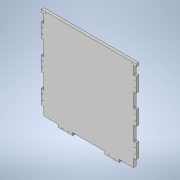
# Autodesk Inventor part: bottom-tool_part
Saved by Autodesk Inventor 2020 (Build 240168000, 168)
## iProperties
Created: 2019-12-17
Part Number: bottom-tool_part
Material: Generic
Document SubType Name: Modeling
Designer: fabfarm
Density: 1 g/cm^3
Appearance: Default
Author: fabfarm
Autodesk Inventor part; units mm, degrees
ref_plane "YZ Plane" through (0, 0, 0) normal (1, 0, 0) x (0, 1, 0)
ref_plane "XZ Plane" through (0, 0, 0) normal (0, 1, 0) x (-1, 0, 0)
ref_plane "XY Plane" through (0, 0, 0) normal (0, 0, 1) x (1, 0, 0)
sketch "Sketch1" plane through (0, 0, 0) normal (0, 0, 1) x (1, 0, 0)
  line L0 (330, -307.45) -> (-330, -307.45)
  line L1 (-330, -307.45) -> (-330, 307.45)
  line L2 (-330, 307.45) -> (330, 307.45)
  line L3 (330, 307.45) -> (330, -307.45)
  line L4 (330, -307.45) -> (-330, 307.45) construction
  line L5 (-330, -307.45) -> (330, 307.45) construction
  point P0 (0, 0)
  dimension "d0" = 614.9
  dimension "d1" = 660
  constraints: 12 end point, 2 midpoint, 2 parallel, 1 horizontal, 1 perpendicular
  measures "d0" distance of L2.end L0.start
  measures "d1" distance of L0.start L0.end
extrude "Extrusion1" add sketch "Sketch1" along normal blind 18.55
sketch "Sketch2" plane through (0, 0, 18.55) normal (0, 0, 1) x (1, 0, 0)
  line L0 (-330, 307.45) -> (-330, -307.45) construction
  line L1 (330, 307.45) -> (-330, 307.45) construction
  line L2 (-330, 307.45) -> (-311.45, 307.45)
  line L3 (-311.45, 307.45) -> (-311.45, 250)
  line L4 (-311.45, 250) -> (-330, 250)
  line L5 (-330, 250) -> (-330, 307.45)
  line L6 (-330, -307.45) -> (330, -307.45) projected
  line L7 (-330, -307.45) -> (-311.45, -307.45)
  line L8 (-311.45, -307.45) -> (-311.45, -250)
  line L9 (-311.45, -250) -> (-330, -250)
  line L10 (-330, -250) -> (-330, -307.45)
  line L11 (-330, -150) -> (-311.45, -150)
  line L12 (-311.45, -150) -> (-311.45, -50)
  line L13 (-311.45, -50) -> (-330, -50)
  line L14 (-330, -50) -> (-330, -150)
  line L15 (-330, 50) -> (-311.45, 50)
  line L16 (-311.45, 50) -> (-311.45, 150)
  line L17 (-311.45, 150) -> (-330, 150)
  line L18 (-330, 150) -> (-330, 50)
  point P0 (0, 0)
  dimension "d21" = 100
  dimension "d22" = 100
  dimension "d23" = 100
  dimension "d24" = 100
  dimension "d25" = 57.45
  dimension "d26" = 18.55
  dimension "d30" = 100
  constraints: 32 end point, 8 parallel, 5 point on line, 4 horizontal, 4 perpendicular, 3 collinear
  measures "d21" distance between parallel lines of L4 L17
  measures "d22" distance of L15.end L16.end
  measures "d23" distance between parallel lines of L13 L15
  measures "d24" distance of L11.end L12.end
  measures "d25" distance of L2.end L3.end
  measures "d26" distance of L0.end L7.end
  measures "d30" distance between parallel lines of L11 L9
extrude "Extrusion2" cut sketch "Sketch2" against normal blind 18.55
mirror "Mirror1" about plane through (0, 0, 0) normal (1, 0, 0) of "Extrusion2"
sketch "Esquisse5" plane through (0, 0, 18.55) normal (0, 0, 1) x (1, 0, 0)
  circle A0 centre (-312.5743, 251.1243) radius 1.59
  circle A1 centre (-312.5743, 148.8757) radius 1.59
  circle A2 centre (-312.5743, 51.1243) radius 1.59
  circle A3 centre (-312.5743, -51.1243) radius 1.59
  circle A4 centre (-312.5743, -148.8757) radius 1.59
  circle A5 centre (-312.5743, -251.1243) radius 1.59
  line L0 (311.45, 307.45) -> (-311.45, 307.45) projected
  line L1 (0, 307.45) -> (0, -307.45) construction
  line L2 (-311.45, -307.45) -> (311.45, -307.45) projected
  circle A6 centre (312.5743, 251.1243) radius 1.59
  circle A7 centre (312.5743, 148.8757) radius 1.59
  circle A8 centre (312.5743, 51.1243) radius 1.59
  circle A9 centre (312.5743, -51.1243) radius 1.59
  circle A10 centre (312.5743, -148.8757) radius 1.59
  circle A11 centre (312.5743, -251.1243) radius 1.59
  line L3 (-312.5743, 251.1243) -> (-311.45, 250) construction
  line L4 (-311.45, 250) -> (-330, 250) projected
  point P0 (0, 0)
  point P1 (-330, 50)
  point P2 (-330, -50)
  point P3 (-311.45, -250)
  point P4 (-311.45, -150)
  point P5 (-311.45, -50)
  point P6 (-311.45, 50)
  point P7 (-311.45, 150)
  dimension "d27" = 3.18
  dimension "d57" = 45
  constraints: 6 centre point, 6 symmetric about line, 5 vertical alignment, 4 end point, 2 midpoint, 24 other
  measures "d57" angle of L3 L4
extrude "Extrusion5" cut sketch "Esquisse5" against normal blind 18.55
sketch "Esquisse7" plane through (0, 0, 18.55) normal (0, 0, 1) x (1, 0, 0)
  line L0 (-311.45, -307.45) -> (311.45, -307.45) projected
  line L1 (-211.45, -307.45) -> (-111.45, -307.45)
  line L2 (-111.45, -307.45) -> (-111.45, -326)
  line L3 (-111.45, -326) -> (-211.45, -326)
  line L4 (-211.45, -326) -> (-211.45, -307.45)
  line L5 (111.55, -307.45) -> (211.45, -307.45)
  line L6 (211.45, -307.45) -> (211.45, -326)
  line L7 (211.45, -326) -> (111.55, -326)
  line L8 (111.55, -326) -> (111.55, -307.45)
  line L9 (-311.45, -252.2486) -> (-311.45, -307.45) projected
  line L10 (311.45, -307.45) -> (311.45, -252.2486) projected
  line L11 (-330, 50) -> (-330, -50) projected
  line L12 (-330, 0) -> (330, 0) construction
  line L13 (330, -50) -> (330, 50) projected
  circle A0 centre (-181.45, -316.725) radius 2.25
  circle A1 centre (-141.45, -316.725) radius 2.25
  circle A2 centre (141.55, -316.725) radius 2.25
  circle A3 centre (181.45, -316.725) radius 2.25
  line L14 (-211.45, -316.725) -> (-111.45, -316.725) construction
  line L15 (311.45, 307.45) -> (-311.45, 307.45) projected
  line L16 (-311.45, 307.45) -> (311.45, 307.45)
  line L17 (311.45, 307.45) -> (311.45, 326)
  line L18 (311.45, 326) -> (-311.45, 326)
  line L19 (-311.45, 326) -> (-311.45, 307.45)
  line L20 (311.45, 252.2486) -> (311.45, 307.45) projected
  point P0 (0, 0)
  point P1 (-111.45, -307.45)
  dimension "d41" = 100
  dimension "d42" = 99.9
  dimension "d43" = 100
  dimension "d44" = 100
  dimension "d45" = 18.55
  dimension "d46" = 4.5
  dimension "d47" = 30
  dimension "d48" = 30
  dimension "d49" = 30
  dimension "d50" = 30
  dimension "d56" = 18.55
  constraints: 28 end point, 7 point on line, 6 parallel, 4 centre point, 4 midpoint, 3 equal radius, 3 horizontal, 3 perpendicular, 1 collinear
  measures "d41" distance of L2.end L3.end
  measures "d42" distance of L6.end L7.end
  measures "d43" distance between parallel lines of L9 L4
  measures "d44" distance between parallel lines of L6 L10
  measures "d45" distance of L1.end L2.end
  measures "d46" diameter of A0
  measures "d47" distance from line of L4 A0.centre
  measures "d48" distance from line of L2 A1.centre
  measures "d49" distance from line of L8 A2.centre
  measures "d50" distance from line of L6 A3.centre
  measures "d56" distance between parallel lines of L18 L15
extrude "Extrusion7" add sketch "Esquisse7" against normal blind 18.55
sketch "Esquisse6" plane through (0, 0, 18.55) normal (0, 0, 1) x (1, 0, 0)
  line L0 (-321.8493, -50) -> (-321.8493, 50) construction
  line L1 (-313.6986, 50) -> (-330, 50) construction
  line L2 (-313.6986, 150) -> (-330, 150) construction
  line L3 (-313.6986, 250) -> (-330, 250) construction
  circle A0 centre (-321.8493, 220) radius 2.25
  line L4 (-330, -50) -> (-313.6986, -50) projected
  line L5 (-0.195, -446.756) -> (0, 307.45) construction
  line L6 (311.45, 307.45) -> (-311.45, 307.45) projected
  line L7 (-321.8493, 150) -> (-321.8493, 250) construction
  circle A1 centre (-321.8493, 180) radius 2.25
  circle A2 centre (-321.8493, 20) radius 2.25
  circle A3 centre (-321.8493, -20) radius 2.25
  line L8 (-313.6986, -150) -> (-330, -150) projected
  line L9 (-321.8493, -150) -> (-321.8493, -250) construction
  line L10 (-313.6986, -250) -> (-330, -250) projected
  circle A4 centre (-321.8493, -180) radius 2.25
  circle A5 centre (-321.8493, -220) radius 2.25
  line L11 (321.6645, -50.1663) -> (321.7162, 49.8336) construction
  line L12 (313.5655, 49.8379) -> (329.8669, 49.8294) construction
  line L13 (313.6172, 149.8378) -> (329.9186, 149.8294) construction
  line L14 (313.6689, 249.8378) -> (329.9703, 249.8294) construction
  circle A6 centre (321.804, 219.8336) radius 2.25
  line L15 (329.8152, -50.1706) -> (313.5138, -50.1621)
  line L16 (321.7679, 149.8336) -> (321.8196, 249.8336) construction
  circle A7 centre (321.7834, 179.8336) radius 2.25
  circle A8 centre (321.7007, 19.8336) radius 2.25
  circle A9 centre (321.68, -20.1663) radius 2.25
  line L17 (313.4621, -150.1621) -> (329.7635, -150.1705)
  line L18 (321.6128, -150.1663) -> (321.5611, -250.1663) construction
  line L19 (313.4104, -250.1621) -> (329.7118, -250.1705)
  circle A10 centre (321.5973, -180.1663) radius 2.25
  circle A11 centre (321.5766, -220.1663) radius 2.25
  point P0 (0, 0)
  dimension "d34" = 30
  dimension "d35" = 30
  dimension "d36" = 30
  dimension "d37" = 30
  dimension "d38" = 4.5
  dimension "d39" = 30
  dimension "d40" = 30
  constraints: 26 end point, 24 symmetric about line, 12 centre point, 12 point on line, 8 midpoint, 5 equal radius, 1 vertical, 6 other
  measures "d34" distance from line of L3 A0.centre
  measures "d35" distance from line of L2 A1.centre
  measures "d36" distance from line of L4 A3.centre
  measures "d37" distance from line of L1 A2.centre
  measures "d38" diameter of A0
  measures "d39" distance from line of L10 A5.centre
  measures "d40" distance from line of L8 A4.centre
extrude "Extrusion6" cut sketch "Esquisse6" against normal blind 20
sketch "Esquisse8" plane through (0, 0, 18.55) normal (0, 0, 1) x (1, 0, 0)
  circle A0 centre (-212.5814, -308.5814) radius 1.6
  circle A1 centre (-110.3186, -308.5814) radius 1.6
  circle A2 centre (110.4186, -308.5814) radius 1.6
  circle A3 centre (212.5814, -308.5814) radius 1.6
  line L0 (211.45, -307.45) -> (212.5814, -308.5814) construction
  line L1 (211.45, -307.45) -> (311.45, -307.45) projected
  point P0 (0, 0)
  point P1 (-111.45, -307.45)
  point P2 (-211.45, -307.45)
  point P3 (111.55, -307.45)
  dimension "d53" = 3.2
  dimension "d58" = 45
  constraints: 3 horizontal alignment, 2 end point, 12 other
  measures "d58" angle of L1 L0
extrude "Extrusion8" cut sketch "Esquisse8" against normal blind 18.55
sketch "Esquisse10" plane through (0, 0, 18.55) normal (0, 0, 1) x (1, 0, 0)
  line L0 (-311.45, 326) -> (-311.45, 252.2486) projected
  line L1 (-311.45, 326) -> (-330, 326)
  line L2 (-330, 326) -> (-330, 307.55)
  line L3 (-330, 307.55) -> (-311.45, 307.55)
  line L4 (-311.45, 307.55) -> (-311.45, 326)
  line L5 (311.45, 326) -> (-311.45, 326) projected
  line L6 (311.45, 326) -> (330, 326)
  line L7 (330, 326) -> (330, 307.55)
  line L8 (330, 307.55) -> (311.45, 307.55)
  line L9 (311.45, 307.55) -> (311.45, 326)
  line L10 (330, 150) -> (330, 250) projected
  line L11 (-330, 250) -> (-330, 150) projected
  point P0 (0, 0)
  dimension "d59" = 18.45
  constraints: 16 end point, 4 parallel, 2 collinear, 2 horizontal, 2 perpendicular, 1 point on line
  measures "d59" distance of L6.end L7.end
extrude "Extrusion9" add sketch "Esquisse10" against normal blind 18.55
sketch "Esquisse11" plane through (0, 0, 18.55) normal (0, 0, 1) x (1, 0, 0)
  line L0 (-311.45, 307.55) -> (-311.45, 252.2486) projected
  circle A0 centre (-312.5814, 306.4186) radius 1.6
  line L1 (311.45, 252.2486) -> (311.45, 307.55) projected
  circle A1 centre (312.5814, 306.4186) radius 1.6
  line L2 (311.45, 307.55) -> (312.5814, 306.4186) construction
  point P0 (0, 0)
  dimension "d63" = 3.2
  dimension "d62" = 45
  constraints: 2 end point, 1 horizontal alignment, 6 other
  measures "d62" angle of L1 L2
extrude "Extrusion10" cut sketch "Esquisse11" against normal blind 20
sketch "Esquisse12" plane through (0, 0, 18.55) normal (0, 0, 1) x (1, 0, 0)
  circle A0 centre (-300, 317.55) radius 2.25
  circle A1 centre (300, 317.55) radius 2.25
  line L0 (-330, 307.55) -> (-313.7127, 307.55) projected
  line L1 (-330, 326) -> (-330, 307.55) projected
  line L2 (330, 307.55) -> (330, 326) projected
  point P0 (0, 0)
  dimension "d66" = 10
  dimension "d67" = 30
  dimension "d68" = 30
  dimension "d69" = 4.5
  constraints: 2 centre point, 1 equal radius, 1 horizontal alignment
  measures "d66" distance from line of L0 A0.centre
  measures "d67" distance from line of L1 A0.centre
  measures "d68" distance from line of L2 A1.centre
  measures "d69" diameter of A1
extrude "Extrusion11" cut sketch "Esquisse12" against normal blind 20
body "Solid1"
